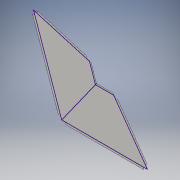
# Autodesk Inventor part: DELL screen 3D hologram piece
Saved by Autodesk Inventor 2016 (Build 200138000, 138)
## iProperties
Created: 2017-09-08
Part Number: DELL screen 3D hologram piece
Material: Generic
Document SubType Name: Modeling
Designer: student
Density: 1 g/cm^3
Appearance: Default
Author: student
Autodesk Inventor part; units mm, degrees
ref_plane "YZ Plane" through (0, 0, 0) normal (1, 0, 0) x (0, 1, 0)
ref_plane "XZ Plane" through (0, 0, 0) normal (0, 1, 0) x (-1, 0, 0)
ref_plane "XY Plane" through (0, 0, 0) normal (0, 0, 1) x (1, 0, 0)
sketch "Sketch1" plane through (0, 0, 0) normal (0, 0, 1) x (1, 0, 0)
  line L0 (-149.2247, -82.55) -> (149.2253, -82.55)
  line L1 (31.75, 82.55) -> (-31.75, 82.55)
  line L2 (31.75, 82.55) -> (149.2253, -82.55)
  line L3 (-31.75, 82.55) -> (-149.2247, -82.55)
  line L4 (-149.2247, -82.55) -> (-247.0638, 199.4073)
  line L5 (-31.75, 82.55) -> (-52.5668, 142.5409)
  line L6 (-247.0638, 199.4073) -> (-52.5668, 142.5409)
  point P0 (0, 0)
  point P1 (0, 82.55)
  point P2 (-90.4873, 0)
  dimension "d1" = 298.45
  dimension "d2" = 63.5
  dimension "d3" = 165.1
  dimension "d4" = 202.6285
  dimension "d5" = 202.6289
  dimension "d31" = 125.433
  dimension "d32" = 125.433
  dimension "d33" = 54.567
  dimension "d34" = 54.567
  dimension "d35" = 54.57
  dimension "d36" = 298.45
  dimension "d37" = 125.43
  dimension "d38" = 63.5
  dimension "d39" = 202.6397
  dimension "d40" = 54.566
  dimension "d41" = 125.434
  constraints: 14 end point, 2 midpoint, 1 horizontal, 1 horizontal alignment, 1 parallel, 1 vertical alignment
  measures "d1" distance of L0.start L0.end
  measures "d2" distance of L1.start L1.end
  measures "d3" distance between parallel lines of L0 L1
  measures "d4" distance of L1.end L0.start
  measures "d5" distance of L1.start L0.end
  measures "d31" angle of L3 L1
  measures "d32" angle of L2 L1
  measures "d33" angle of L0 L2
  measures "d34" angle of L0 L3
  measures "d35" angle of L4 L3
  measures "d36" distance of L0.start L4.end
  measures "d37" angle of L3 L5
  measures "d38" distance of L1.end L5.end
  measures "d39" distance of L4.end L5.end
  measures "d40" angle of L4 L6
  measures "d41" angle of L5 L6
extrude "Extrusion2" add sketch "Sketch1" along normal blind 0.127
sketch "Sketch3" plane through (0, 0, 0.127) normal (0, 0, 1) x (1, 0, 0)
  line L0 (31.75, 82.55) -> (-31.75, 82.55) projected
  line L1 (-31.75, 82.55) -> (31.75, 82.55)
  line L2 (-31.75, 82.55) -> (-28.1358, 87.63)
  line L3 (31.75, 82.55) -> (28.1358, 87.63)
  line L4 (-28.1358, 87.63) -> (28.1358, 87.63)
  line L5 (-31.75, 82.55) -> (-52.5668, 142.5409) projected
  line L6 (-52.5668, 142.5409) -> (-46.5827, 140.7918)
  line L7 (-46.5827, 140.7918) -> (-28.1358, 87.63)
  line L8 (-149.2247, -82.55) -> (149.2253, -82.55) projected
  line L9 (-52.5668, 142.5409) -> (-247.0638, 199.4073) projected
  line L10 (-247.0638, 199.4073) -> (-149.2247, -82.55) projected
  line L11 (136.5253, -90.17) -> (-136.5247, -90.17)
  line L12 (-247.0638, 199.4073) -> (-149.2247, -82.55) projected
  line L13 (-160.5869, -73.0498) -> (-250.0993, 184.9111)
  line L14 (-232.7357, 203.1571) -> (-62.6181, 153.4187)
  line L15 (-31.75, 82.55) -> (31.75, 82.55)
  line L16 (149.2253, -82.55) -> (31.75, 82.55) projected
  line L17 (45.3216, 76.6199) -> (148.0711, -67.7844)
  line L18 (31.75, 82.55) -> (149.2253, -82.55)
  line L19 (-52.5668, 142.5409) -> (-31.75, 82.55)
  line L20 (-46.5827, 140.7918) -> (-28.1358, 87.63)
  line L21 (-28.1358, 87.63) -> (28.1358, 87.63)
  line L22 (-232.7357, 203.1571) -> (-234.8741, 195.8433)
  line L23 (-64.7565, 146.1049) -> (-62.6181, 153.4187)
  line L24 (-250.0993, 184.9111) -> (-242.9004, 187.4091)
  line L25 (-160.5869, -73.0498) -> (-153.388, -70.5518)
  line L26 (-136.5247, -82.55) -> (-136.5247, -90.17)
  line L27 (136.5253, -82.55) -> (136.5253, -90.17)
  line L28 (148.0711, -67.7844) -> (141.8624, -72.2022)
  line L29 (45.3216, 76.6199) -> (39.1129, 72.2022)
  point P0 (0, 0)
  dimension "d45" = 54.57
  dimension "d46" = 5.08
  dimension "d47" = 54.57
  dimension "d48" = 54.57
  dimension "d51" = 5.08
  dimension "d68" = 7.62
  dimension "d84" = 7.62
  dimension "d89" = 90
  dimension "d90" = 12.7
  dimension "d91" = 7.62
  dimension "d93" = 90
  dimension "d94" = 12.7
  dimension "d95" = 12.7
  dimension "d97" = 12.7
  dimension "d98" = 90
  dimension "d99" = 90
  dimension "d100" = 7.62
  dimension "d101" = 12.7
  dimension "d102" = 12.7
  dimension "d103" = 7.62
  dimension "d104" = 7.62
  dimension "d105" = 12.7
  dimension "d106" = 12.7
  dimension "d107" = 7.62
  dimension "d108" = 7.62
  dimension "d109" = 90
  constraints: 46 end point, 8 point on line, 7 perpendicular, 3 horizontal, 2 parallel, 1 collinear
  measures "d45" angle of L0 L2
  measures "d46" distance from line of L2.end L0
  measures "d47" angle of L0 L3
  measures "d48" angle of L5 L6
  measures "d51" distance from line of L5 L6.end
  measures "d68" distance from line of L10 L13.end
  measures "d84" distance from line of L10 L13.start
  measures "d89" angle of L9 L22
  measures "d90" distance from line of L9.end L22
  measures "d91" distance between parallel lines of L9 L14
  measures "d93" angle of L9 L23
  measures "d94" distance from line of L5.end L23
  measures "d95" distance from line of L9.end L24
  measures "d97" distance from line of L25 L8.start
  measures "d98" angle of L10 L25
  measures "d99" angle of L10 L24
  measures "d100" distance of L23.start L14.end
  measures "d101" distance from line of L8.end L27
  measures "d102" distance from line of L8.start L26
  measures "d103" distance between parallel lines of L8 L11
  measures "d104" distance of L27.start L11.start
  measures "d105" distance from line of L0.start L29
  measures "d106" distance from line of L8.end L28
  measures "d107" distance of L17.start L29.end
  measures "d108" distance between parallel lines of L16 L17
  measures "d109" angle of L16 L28
extrude "Extrusion4" add sketch "Sketch3" along normal blind 0.127
sketch "Sketch5" plane through (0, 0, 0.254) normal (0, 0, 1) x (1, 0, 0)
  line L0 (31.75, 82.55) -> (-31.75, 82.55) projected
  line L1 (31.75, 82.55) -> (-31.75, 82.55)
  line L2 (-149.2247, -82.55) -> (149.2253, -82.55) projected
  line L3 (31.75, 82.55) -> (149.2253, -82.55)
  line L4 (149.2253, -82.55) -> (-149.2247, -82.55)
  line L5 (-242.9004, 187.4091) -> (-149.2247, -82.55) projected
  line L6 (-149.2247, -82.55) -> (-247.0638, 199.4073)
  line L7 (-247.0638, 199.4073) -> (-52.5668, 142.5409)
  line L8 (-31.75, 82.55) -> (-52.5668, 142.5409) projected
  line L9 (-52.5668, 142.5409) -> (-31.75, 82.55)
  line L10 (-31.75, 82.55) -> (-28.1358, 87.63)
  line L11 (-31.75, 82.55) -> (-149.2247, -82.55)
  constraints: 16 end point, 3 collinear, 1 horizontal
body "Solid2"
